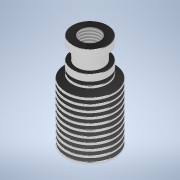
# Autodesk Inventor part: v6-hotend-heatsink
Saved by Autodesk Inventor 2021 (Build 250183000, 183)
## iProperties
Created: 2021-01-15
Part Number: v6-hotend-heatsink
Material: Aluminum 6061
Document SubType Name: Modeling
Designer: WubbGmbaa
Density: 2.7 g/cm^3
Appearance: Chrome - Polished
Author: WubbGmbaa
Autodesk Inventor part; units mm, degrees
ref_plane "YZ Plane" through (0, 0, 0) normal (1, 0, 0) x (0, 1, 0)
ref_plane "XZ Plane" through (0, 0, 0) normal (0, 1, 0) x (-1, 0, 0)
ref_plane "XY Plane" through (0, 0, 0) normal (0, 0, 1) x (1, 0, 0)
sketch "Sketch1" plane through (0, 0, 0) normal (0, 0, 1) x (1, 0, 0)
  line L0 (0, 0) -> (11.07, 0) construction
  line L1 (11.07, 0) -> (11.07, 26.11) construction
  line L2 (11.07, 26.11) -> (0, 26.11) construction
  line L3 (0, 26.11) -> (0, 0) construction
  line L4 (0, 26.11) -> (8, 26.11) construction
  line L5 (8, 26.11) -> (8, 42.81) construction
  line L6 (8, 42.81) -> (0, 42.81) construction
  line L7 (0, 42.81) -> (0, 26.11) construction
  line L8 (8, 42.81) -> (0, 42.81) construction
  line L9 (0, 42.81) -> (0, 30.16) construction
  line L10 (0, 30.16) -> (8, 30.16) construction
  line L11 (8, 30.16) -> (8, 42.81) construction
  line L12 (0, 42.81) -> (8, 42.81) construction
  line L13 (8, 42.81) -> (8, 39.206) construction
  line L14 (8, 39.206) -> (0, 39.206) construction
  line L15 (0, 39.206) -> (0, 42.81) construction
  line L16 (0, 39.206) -> (8, 39.206) construction
  line L17 (8, 39.206) -> (8, 33.206) construction
  line L18 (8, 33.206) -> (0, 33.206) construction
  line L19 (0, 33.206) -> (0, 39.206) construction
  line L20 (0, 39.206) -> (6, 39.206) construction
  line L21 (6, 39.206) -> (6, 33.206) construction
  line L22 (6, 33.206) -> (0, 33.206) construction
  line L23 (0, 33.206) -> (0, 39.206) construction
  line L24 (0, 30.16) -> (8, 30.16) construction
  line L25 (8, 30.16) -> (8, 28.59) construction
  line L26 (8, 28.59) -> (0, 28.59) construction
  line L27 (0, 28.59) -> (0, 30.16) construction
  line L28 (0, 28.59) -> (8, 28.59) construction
  line L29 (8, 28.59) -> (8, 27.55) construction
  line L30 (8, 27.55) -> (0, 27.55) construction
  line L31 (0, 27.55) -> (0, 28.59) construction
  line L32 (0, 42.81) -> (4.45, 42.81) construction
  line L33 (4.45, 42.81) -> (4.45, 31.26) construction
  line L34 (4.45, 31.26) -> (0, 31.26) construction
  line L35 (0, 31.26) -> (0, 42.81) construction
  line L36 (0, 0) -> (6.1, 0) construction
  line L37 (6.1, 0) -> (6.1, 15.42) construction
  line L38 (6.1, 15.42) -> (0, 15.42) construction
  line L39 (0, 15.42) -> (0, 0) construction
  line L40 (0, 31.26) -> (2.1, 31.26) construction
  line L41 (2.1, 31.26) -> (2.1, 15.42) construction
  line L42 (2.1, 15.42) -> (0, 15.42) construction
  line L43 (0, 15.42) -> (0, 31.26) construction
  line L44 (0, 15.42) -> (3.05, 15.42) construction
  line L45 (3.05, 15.42) -> (3.05, 0) construction
  line L46 (3.05, 0) -> (0, 0) construction
  line L47 (0, 0) -> (0, 15.42) construction
  line L48 (3.05, 0) -> (3.05, 15.42)
  line L49 (3.05, 15.42) -> (2.1, 15.42)
  line L50 (2.1, 15.42) -> (2.1, 31.26)
  line L51 (2.1, 31.26) -> (4.45, 31.26)
  line L52 (4.45, 31.26) -> (4.45, 42.81)
  line L53 (4.45, 42.81) -> (8, 42.81)
  line L54 (8, 42.81) -> (8, 39.206)
  line L55 (8, 39.206) -> (6, 39.206)
  line L56 (6, 39.206) -> (6, 33.206)
  line L57 (6, 33.206) -> (8, 33.206)
  line L58 (8, 33.206) -> (8, 30.16)
  line L59 (8, 30.16) -> (4.46, 30.16) construction
  line L60 (4.46, 30.16) -> (4.46, 26.11) construction
  line L61 (4.46, 26.11) -> (8, 26.11) construction
  line L62 (8, 26.11) -> (8, 30.16) construction
  line L63 (8, 30.16) -> (4.46, 30.16) construction
  line L64 (8, 30.16) -> (4.46, 30.16)
  line L65 (4.46, 30.16) -> (4.46, 28.59)
  line L66 (4.46, 28.59) -> (8, 28.59)
  line L67 (8, 28.59) -> (8, 27.55)
  line L68 (8, 27.55) -> (4.46, 27.55)
  line L69 (4.46, 27.55) -> (4.46, 26.11)
  line L70 (4.46, 26.11) -> (11.07, 26.11)
  line L71 (3.05, 0) -> (11.07, 0)
  line L72 (11.07, 26.11) -> (4.65, 26.11) construction
  line L73 (11.07, 0) -> (6.24, 0) construction
  line L74 (6.24, 0) -> (4.65, 26.11) construction
  line L75 (11.07, 26.11) -> (2.1, 26.11) construction
  line L76 (2.1, 26.11) -> (2.1, 25.04) construction
  line L77 (2.1, 25.04) -> (11.07, 25.04) construction
  line L78 (11.07, 25.04) -> (11.07, 26.11) construction
  line L79 (3.05, 0) -> (11.07, 0) construction
  line L80 (11.07, 0) -> (11.07, 2.504) construction
  line L81 (11.07, 2.504) -> (3.05, 2.504) construction
  line L82 (3.05, 2.504) -> (3.05, 0) construction
  line L83 (11.07, 0) -> (3.05, 0) construction
  line L84 (3.05, 0) -> (3.05, 1.04) construction
  line L85 (3.05, 1.04) -> (11.07, 1.04) construction
  line L86 (11.07, 1.04) -> (11.07, 0) construction
  line L87 (11.07, 0) -> (11.07, 1.04)
  line L88 (11.07, 2.504) -> (11.07, 3.544)
  line L89 (11.07, 5.008) -> (11.07, 6.048)
  line L90 (11.07, 7.512) -> (11.07, 8.552)
  line L91 (11.07, 10.016) -> (11.07, 11.056)
  line L92 (11.07, 12.52) -> (11.07, 13.56)
  line L93 (11.07, 15.024) -> (11.07, 16.064)
  line L94 (11.07, 17.528) -> (11.07, 18.568)
  line L95 (11.07, 20.032) -> (11.07, 21.072)
  line L96 (11.07, 22.536) -> (11.07, 23.576)
  line L97 (11.07, 26.11) -> (11.07, 25.04)
  line L98 (11.07, 25.04) -> (4.7152, 25.04)
  line L99 (4.7152, 25.04) -> (4.8043, 23.576)
  line L100 (4.8676, 22.536) -> (4.9568, 21.072)
  line L101 (5.0201, 20.032) -> (5.1093, 18.568)
  line L102 (5.1726, 17.528) -> (5.2618, 16.064)
  line L103 (5.3251, 15.024) -> (5.4142, 13.56)
  line L104 (5.4776, 12.52) -> (5.5667, 11.056)
  line L105 (5.6301, 10.016) -> (5.7192, 8.552)
  line L106 (5.7825, 7.512) -> (5.8717, 6.048)
  line L107 (5.935, 5.008) -> (6.0242, 3.544)
  line L108 (6.0875, 2.504) -> (6.1767, 1.04)
  line L109 (6.1767, 1.04) -> (11.07, 1.04)
  line L110 (6.0875, 2.504) -> (11.07, 2.504)
  line L111 (11.07, 3.544) -> (6.0242, 3.544)
  line L112 (5.935, 5.008) -> (11.07, 5.008)
  line L113 (11.07, 6.048) -> (5.8717, 6.048)
  line L114 (5.7825, 7.512) -> (11.07, 7.512)
  line L115 (11.07, 8.552) -> (5.7192, 8.552)
  line L116 (5.6301, 10.016) -> (11.07, 10.016)
  line L117 (11.07, 11.056) -> (5.5667, 11.056)
  line L118 (5.4776, 12.52) -> (11.07, 12.52)
  line L119 (11.07, 13.56) -> (5.4142, 13.56)
  line L120 (5.3251, 15.024) -> (11.07, 15.024)
  line L121 (11.07, 16.064) -> (5.2618, 16.064)
  line L122 (5.1726, 17.528) -> (11.07, 17.528)
  line L123 (11.07, 18.568) -> (5.1093, 18.568)
  line L124 (5.0201, 20.032) -> (11.07, 20.032)
  line L125 (11.07, 21.072) -> (4.9568, 21.072)
  line L126 (4.8676, 22.536) -> (11.07, 22.536)
  line L127 (11.07, 23.576) -> (4.8043, 23.576)
  dimension "d9" = 11.07
  dimension "d10" = 26.11
  dimension "d11" = 8
  dimension "d12" = 16.7
  dimension "d13" = 8
  dimension "d14" = 12.65
  dimension "d15" = 6
  dimension "d16" = 6
  dimension "d17" = 1.57
  dimension "d18" = 8
  dimension "d19" = 1.04
  dimension "d20" = 4.45
  dimension "d21" = 11.55
  dimension "d22" = 6.1
  dimension "d23" = 15.42
  dimension "d24" = 2.1
  dimension "d25" = 3.05
  dimension "d26" = 3.54
  dimension "d27" = 6.42
  dimension "d28" = 4.83
  dimension "d29" = 1.07
  dimension "d30" = 2.504
  dimension "d31" = 1.04
  dimension "d34" = 2.504
  constraints: 254 end point, 47 parallel, 24 perpendicular, 18 point on line, 17 horizontal, 12 collinear, 3 vertical, 1 midpoint, 50 other
  measures "d9" distance of L2.end L1.end
  measures "d10" distance of L1.end L0.end
  measures "d11" distance of L6.end L5.end
  measures "d12" distance of L5.end L4.end
  measures "d13" distance of L10.end L9.end
  measures "d14" distance of L9.end L8.end
  measures "d15" distance of L16.end L17.end
  measures "d16" distance of L21.end L22.end
  measures "d17" distance of L24.end L25.end
  measures "d18" distance of L29.end L30.end
  measures "d19" distance of L28.end L29.end
  measures "d20" distance of L33.end L34.end
  measures "d21" distance of L32.end L33.end
  measures "d22" distance of L38.end L37.end
  measures "d23" distance of L37.end L36.end
  measures "d24" distance of L41.end L42.end
  measures "d25" distance of L45.end L46.end
  measures "d26" distance of L61.end L60.end
  measures "d27" distance of L1.end L72.end
  measures "d28" distance of L0.end L73.end
  measures "d29" distance of L76.end L75.end
  measures "d30" distance of L80.end L79.end
  measures "d31" distance of L83.end L84.end
  measures "d34" distance of L79.end L88.start
revolve "Revolution1" add sketch "Sketch1" angle 360 about axis through (0, 33.206, 0) along (0, 1, 0)
fillet "Fillet1" radius 0.25 24 edges at (-11.07, 26.11, 0) (-11.07, 25.04, 0) (-11.07, 23.576, 0) (-11.07, 22.536, 0) (-8, 27.55, 0) (-8, 28.59, 0) (-11.07, 21.072, 0) (-11.07, 20.032, 0) (-11.07, 18.568, 0) (-11.07, 17.528, 0) (-11.07, 16.064, 0) (-11.07, 15.024, 0) (-11.07, 13.56, 0) (-11.07, 12.52, 0) (-11.07, 11.056, 0) (-11.07, 10.016, 0) (-11.07, 8.552, 0) (-11.07, 7.512, 0) (-11.07, 6.048, 0) (-11.07, 5.008, 0) (-11.07, 3.544, 0) (-11.07, 2.504, 0) (-11.07, 1.04, 0) (-11.07, 0, 0)
fillet "Fillet2" radius 0.25 5 edges at (-8, 42.81, 0) (-8, 39.206, 0) (-8, 33.206, 0) (-8, 30.16, 0) (-3.05, 0, 0)
thread "Thread1" size "M7x1" class "6H" standard "ANSI Metric M Profile" full length
thread "Thread2" size "M9x1.25" class "6H" standard "ANSI Metric M Profile" full length
body "Solid1"
